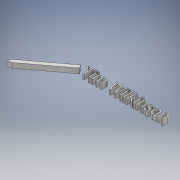
# Autodesk Inventor part: Tim
Saved by Autodesk Inventor 2017 (Build 210142000, 142)
## iProperties
Created: 2021-02-26
Part Number: Tim
Material: Generic
Document SubType Name: Modeling
Designer: paulg
Density: 1 g/cm^3
Appearance: Default
Author: paulg
Autodesk Inventor part; units mm, degrees
ref_plane "YZ Plane" through (0, 0, 0) normal (1, 0, 0) x (0, 1, 0)
ref_plane "XZ Plane" through (0, 0, 0) normal (0, 1, 0) x (-1, 0, 0)
ref_plane "XY Plane" through (0, 0, 0) normal (0, 0, 1) x (1, 0, 0)
sketch "Sketch1" plane through (0, 0, 0) normal (0, 0, 1) x (1, 0, 0)
  line L0 (-0.0217, 0.1086) -> (95.9171, 0.1086) construction
  line L1 (95.9171, 0.1086) -> (95.9171, -3.6211) construction
  line L2 (95.9171, -3.6211) -> (-0.0217, -3.6211) construction
  line L3 (-0.0217, -3.6211) -> (-0.0217, 0.1086) construction
  line L4 (-41.7116, -36.1087) -> (-2.9577, -7.16)
  line L5 (-2.9577, -7.16) -> (-5.3043, -4.0186)
  line L6 (-5.3043, -4.0186) -> (-44.0582, -32.9673)
  line L7 (-44.0582, -32.9673) -> (-41.7116, -36.1087)
  line L8 (-41.7116, -36.1087) -> (-5.3043, -4.0186) construction
  line L9 (-2.9577, -7.16) -> (-44.0582, -32.9673) construction
  line L10 (-44.0582, -32.9673) -> (-46.1916, -37.008)
  line L11 (-46.1916, -37.008) -> (-41.7116, -36.1087)
  line L12 (-46.1916, -37.008) -> (-42.8849, -34.538) construction
  line L13 (3.3251, -10.3371) -> (3.3251, -1.5202)
  line L14 (3.3251, -1.5202) -> (-0.0298, -1.5202)
  line L15 (-0.0298, -1.5202) -> (-0.0298, -0.3371)
  line L16 (-0.0298, -0.3371) -> (8.0091, -0.3371)
  line L17 (8.0091, -0.3371) -> (8.0091, -1.5202)
  line L18 (8.0091, -1.5202) -> (4.6541, -1.5202)
  line L19 (4.6541, -1.5202) -> (4.6541, -10.3371)
  line L20 (4.6541, -10.3371) -> (3.3251, -10.3371)
  line L21 (10.2133, -10.3371) -> (8.9491, -10.3371)
  line L22 (8.9491, -10.3371) -> (8.9491, -2.833)
  line L23 (8.9491, -2.833) -> (10.2133, -2.833)
  line L24 (10.2133, -2.833) -> (10.2133, -10.3371)
  line L25 (10.3024, -1.585) -> (8.8681, -1.585)
  line L26 (8.8681, -1.585) -> (8.8681, -0.2722)
  line L27 (8.8681, -0.2722) -> (10.3024, -0.2722)
  line L28 (10.3024, -0.2722) -> (10.3024, -1.585)
  line L29 (20.5779, -10.3371) -> (20.5779, -5.9935)
  spline S0 degree 2 poles (20.5779, -5.9935) (20.5779, -5.4748) (20.4969, -4.5915) (20.3672, -4.3484) knots 0 0 0 1 2 2 2
  spline S1 degree 2 poles (20.3672, -4.3484) (20.2376, -4.081) (19.7433, -3.8217) (19.3138, -3.8217) knots 0 0 0 1 2 2 2
  spline S2 degree 2 poles (19.3138, -3.8217) (18.9248, -3.8217) (18.0334, -4.2998) (17.5634, -4.7536) knots 0 0 0 1 2 2 2
  spline S3 degree 2 poles (17.5634, -4.7536) (17.5715, -4.867) (17.5877, -5.1831) (17.5877, -5.3938) knots 0 0 0 1 2 2 2
  line L30 (17.5877, -5.3938) -> (17.5877, -10.3371)
  line L31 (17.5877, -10.3371) -> (16.3235, -10.3371)
  line L32 (16.3235, -10.3371) -> (16.3235, -5.9935)
  spline S4 degree 2 poles (16.3235, -5.9935) (16.3235, -5.4748) (16.2425, -4.5915) (16.1128, -4.3484) knots 0 0 0 1 2 2 2
  spline S5 degree 2 poles (16.1128, -4.3484) (15.9831, -4.081) (15.4888, -3.8217) (15.0593, -3.8217) knots 0 0 0 1 2 2 2
  spline S6 degree 2 poles (15.0593, -3.8217) (14.6541, -3.8217) (13.7546, -4.3322) (13.3332, -4.7293) knots 0 0 0 1 2 2 2
  line L33 (13.3332, -4.7293) -> (13.3332, -10.3371)
  line L34 (13.3332, -10.3371) -> (12.069, -10.3371)
  line L35 (12.069, -10.3371) -> (12.069, -2.833)
  line L36 (12.069, -2.833) -> (13.3332, -2.833)
  line L37 (13.3332, -2.833) -> (13.3332, -3.6596)
  spline S7 degree 2 poles (13.3332, -3.6596) (13.8275, -3.1653) (14.8, -2.6223) (15.3835, -2.6223) knots 0 0 0 1 2 2 2
  spline S8 degree 2 poles (15.3835, -2.6223) (16.048, -2.6223) (17.0771, -3.2301) (17.3446, -3.9189) knots 0 0 0 1 2 2 2
  spline S9 degree 2 poles (17.3446, -3.9189) (17.9199, -3.2787) (19.0058, -2.6223) (19.6379, -2.6223) knots 0 0 0 1 2 2 2
  spline S10 degree 2 poles (19.6379, -2.6223) (20.1241, -2.6223) (20.9183, -2.9221) (21.21, -3.2625) knots 0 0 0 1 2 2 2
  spline S11 degree 2 poles (21.21, -3.2625) (21.5099, -3.6029) (21.8421, -4.6239) (21.8421, -5.3938) knots 0 0 0 1 2 2 2
  line L38 (21.8421, -5.3938) -> (21.8421, -10.3371)
  line L39 (21.8421, -10.3371) -> (20.5779, -10.3371)
  line L40 (39.2165, -0.3371) -> (36.7044, -10.3371)
  line L41 (36.7044, -10.3371) -> (35.2133, -10.3371)
  line L42 (35.2133, -10.3371) -> (33.1792, -2.0388)
  line L43 (33.1792, -2.0388) -> (31.2019, -10.3371)
  line L44 (31.2019, -10.3371) -> (29.7271, -10.3371)
  line L45 (29.7271, -10.3371) -> (27.1744, -0.3371)
  line L46 (27.1744, -0.3371) -> (28.5439, -0.3371)
  line L47 (28.5439, -0.3371) -> (30.5536, -8.6272)
  line L48 (30.5536, -8.6272) -> (32.5472, -0.3371)
  line L49 (32.5472, -0.3371) -> (33.9005, -0.3371)
  line L50 (33.9005, -0.3371) -> (35.9102, -8.7244)
  line L51 (35.9102, -8.7244) -> (37.9118, -0.3371)
  line L52 (37.9118, -0.3371) -> (39.2165, -0.3371)
  line L53 (41.599, -10.3371) -> (40.3348, -10.3371)
  line L54 (40.3348, -10.3371) -> (40.3348, -2.833)
  line L55 (40.3348, -2.833) -> (41.599, -2.833)
  line L56 (41.599, -2.833) -> (41.599, -10.3371)
  line L57 (41.6882, -1.585) -> (40.2538, -1.585)
  line L58 (40.2538, -1.585) -> (40.2538, -0.2722)
  line L59 (40.2538, -0.2722) -> (41.6882, -0.2722)
  line L60 (41.6882, -0.2722) -> (41.6882, -1.585)
  line L61 (44.7433, -10.3371) -> (43.4791, -10.3371)
  line L62 (43.4791, -10.3371) -> (43.4791, 0.1086)
  line L63 (43.4791, 0.1086) -> (44.7433, 0.1086)
  line L64 (44.7433, 0.1086) -> (44.7433, -10.3371)
  line L65 (52.8146, -10.3371) -> (51.1533, -10.3371)
  line L66 (51.1533, -10.3371) -> (48.3656, -6.7147)
  line L67 (48.3656, -6.7147) -> (47.8632, -7.2009)
  line L68 (47.8632, -7.2009) -> (47.8632, -10.3371)
  line L69 (47.8632, -10.3371) -> (46.599, -10.3371)
  line L70 (46.599, -10.3371) -> (46.599, 0.1086)
  line L71 (46.599, 0.1086) -> (47.8632, 0.1086)
  line L72 (47.8632, 0.1086) -> (47.8632, -6.0016)
  line L73 (47.8632, -6.0016) -> (50.8292, -2.833)
  line L74 (50.8292, -2.833) -> (52.4013, -2.833)
  line L75 (52.4013, -2.833) -> (49.3219, -5.9692)
  line L76 (49.3219, -5.9692) -> (52.8146, -10.3371)
  line L77 (54.7352, -10.3371) -> (53.471, -10.3371)
  line L78 (53.471, -10.3371) -> (53.471, -2.833)
  line L79 (53.471, -2.833) -> (54.7352, -2.833)
  line L80 (54.7352, -2.833) -> (54.7352, -10.3371)
  line L81 (54.8243, -1.585) -> (53.3899, -1.585)
  line L82 (53.3899, -1.585) -> (53.3899, -0.2722)
  line L83 (53.3899, -0.2722) -> (54.8243, -0.2722)
  line L84 (54.8243, -0.2722) -> (54.8243, -1.585)
  line L85 (62.4823, -10.3371) -> (61.2181, -10.3371)
  line L86 (61.2181, -10.3371) -> (61.2181, -6.0583)
  spline S12 degree 2 poles (61.2181, -6.0583) (61.2181, -5.5397) (61.1209, -4.6482) (60.975, -4.3808) knots 0 0 0 1 2 2 2
  spline S13 degree 2 poles (60.975, -4.3808) (60.8211, -4.0972) (60.27, -3.8217) (59.8, -3.8217) knots 0 0 0 1 2 2 2
  spline S14 degree 2 poles (59.8, -3.8217) (59.33, -3.8217) (58.3332, -4.3241) (57.8551, -4.7293) knots 0 0 0 1 2 2 2
  line L87 (57.8551, -4.7293) -> (57.8551, -10.3371)
  line L88 (57.8551, -10.3371) -> (56.5909, -10.3371)
  line L89 (56.5909, -10.3371) -> (56.5909, -2.833)
  line L90 (56.5909, -2.833) -> (57.8551, -2.833)
  line L91 (57.8551, -2.833) -> (57.8551, -3.6677)
  spline S15 degree 2 poles (57.8551, -3.6677) (58.4224, -3.1572) (59.5164, -2.6223) (60.1322, -2.6223) knots 0 0 0 1 2 2 2
  spline S16 degree 2 poles (60.1322, -2.6223) (61.2343, -2.6223) (62.4823, -4.081) (62.4823, -5.4667) knots 0 0 0 1 2 2 2
  line L92 (62.4823, -5.4667) -> (62.4823, -10.3371)
  spline S17 degree 2 poles (66.283, -10.5153) (65.5293, -10.5153) (64.2246, -10.1102) (63.7951, -9.8833) knots 0 0 0 1 2 2 2
  line L93 (63.7951, -9.8833) -> (63.7951, -8.4651)
  line L94 (63.7951, -8.4651) -> (63.86, -8.4651)
  spline S18 degree 2 poles (63.86, -8.4651) (64.022, -8.5948) (64.4596, -8.9027) (64.8243, -9.0729) knots 0 0 0 1 2 2 2
  spline S19 degree 2 poles (64.8243, -9.0729) (65.1403, -9.2268) (65.9183, -9.4538) (66.3316, -9.4538) knots 0 0 0 1 2 2 2
  spline S20 degree 2 poles (66.3316, -9.4538) (66.6314, -9.4538) (67.3202, -9.316) (67.4823, -9.2025) knots 0 0 0 1 2 2 2
  spline S21 degree 2 poles (67.4823, -9.2025) (67.7173, -9.0486) (67.928, -8.7001) (67.928, -8.3435) knots 0 0 0 1 2 2 2
  spline S22 degree 2 poles (67.928, -8.3435) (67.928, -7.8978) (67.4418, -7.4359) (66.8178, -7.282) knots 0 0 0 1 2 2 2
  spline S23 degree 2 poles (66.8178, -7.282) (66.5747, -7.2252) (65.7967, -7.0632) (65.4645, -6.974) knots 0 0 0 1 2 2 2
  spline S24 degree 2 poles (65.4645, -6.974) (64.6055, -6.7228) (63.8275, -5.6855) (63.8275, -4.9481) knots 0 0 0 1 2 2 2
  spline S25 degree 2 poles (63.8275, -4.9481) (63.8275, -3.927) (65.3591, -2.6547) (66.6233, -2.6547) knots 0 0 0 1 2 2 2
  spline S26 degree 2 poles (66.6233, -2.6547) (67.2473, -2.6547) (68.5115, -2.9627) (68.941, -3.1977) knots 0 0 0 1 2 2 2
  line L95 (68.941, -3.1977) -> (68.941, -4.551)
  line L96 (68.941, -4.551) -> (68.8762, -4.551)
  spline S27 degree 2 poles (68.8762, -4.551) (68.3899, -4.162) (67.2068, -3.7163) (66.599, -3.7163) knots 0 0 0 1 2 2 2
  spline S28 degree 2 poles (66.599, -3.7163) (65.975, -3.7163) (65.116, -4.2431) (65.116, -4.7698) knots 0 0 0 1 2 2 2
  spline S29 degree 2 poles (65.116, -4.7698) (65.116, -5.2479) (65.6266, -5.7098) (66.1938, -5.8557) knots 0 0 0 1 2 2 2
  spline S30 degree 2 poles (66.1938, -5.8557) (66.4694, -5.9286) (67.1663, -6.0745) (67.5472, -6.1636) knots 0 0 0 1 2 2 2
  spline S31 degree 2 poles (67.5472, -6.1636) (68.3737, -6.3743) (69.2165, -7.3387) (69.2165, -8.1734) knots 0 0 0 1 2 2 2
  spline S32 degree 2 poles (69.2165, -8.1734) (69.2165, -8.6596) (68.8356, -9.5186) (68.4629, -9.8346) knots 0 0 0 1 2 2 2
  spline S33 degree 2 poles (68.4629, -9.8346) (68.0658, -10.1669) (67.0528, -10.5153) (66.283, -10.5153) knots 0 0 0 1 2 2 2
  spline S34 degree 2 poles (76.5585, -6.585) (76.5585, -8.4813) (74.7352, -10.5478) (73.2117, -10.5478) knots 0 0 0 1 2 2 2
  spline S35 degree 2 poles (73.2117, -10.5478) (71.6476, -10.5478) (69.8567, -8.4165) (69.8567, -6.585) knots 0 0 0 1 2 2 2
  spline S36 degree 2 poles (69.8567, -6.585) (69.8567, -4.705) (71.7044, -2.6223) (73.2117, -2.6223) knots 0 0 0 1 2 2 2
  spline S37 degree 2 poles (73.2117, -2.6223) (74.7352, -2.6223) (76.5585, -4.6969) (76.5585, -6.585) knots 0 0 0 1 2 2 2
  spline S38 degree 2 poles (75.2538, -6.585) (75.2538, -5.1264) (74.1922, -3.7082) (73.2117, -3.7082) knots 0 0 0 1 2 2 2
  spline S39 degree 2 poles (73.2117, -3.7082) (72.2311, -3.7082) (71.1614, -5.1264) (71.1614, -6.585) knots 0 0 0 1 2 2 2
  spline S40 degree 2 poles (71.1614, -6.585) (71.1614, -8.0032) (72.2311, -9.4619) (73.2117, -9.4619) knots 0 0 0 1 2 2 2
  spline S41 degree 2 poles (73.2117, -9.4619) (74.1841, -9.4619) (75.2538, -8.0275) (75.2538, -6.585) knots 0 0 0 1 2 2 2
  line L97 (83.7465, -10.3371) -> (82.4823, -10.3371)
  line L98 (82.4823, -10.3371) -> (82.4823, -6.0583)
  spline S42 degree 2 poles (82.4823, -6.0583) (82.4823, -5.5397) (82.3851, -4.6482) (82.2392, -4.3808) knots 0 0 0 1 2 2 2
  spline S43 degree 2 poles (82.2392, -4.3808) (82.0852, -4.0972) (81.5342, -3.8217) (81.0642, -3.8217) knots 0 0 0 1 2 2 2
  spline S44 degree 2 poles (81.0642, -3.8217) (80.5942, -3.8217) (79.5974, -4.3241) (79.1193, -4.7293) knots 0 0 0 1 2 2 2
  line L99 (79.1193, -4.7293) -> (79.1193, -10.3371)
  line L100 (79.1193, -10.3371) -> (77.8551, -10.3371)
  line L101 (77.8551, -10.3371) -> (77.8551, -2.833)
  line L102 (77.8551, -2.833) -> (79.1193, -2.833)
  line L103 (79.1193, -2.833) -> (79.1193, -3.6677)
  spline S45 degree 2 poles (79.1193, -3.6677) (79.6865, -3.1572) (80.7805, -2.6223) (81.3964, -2.6223) knots 0 0 0 1 2 2 2
  spline S46 degree 2 poles (81.3964, -2.6223) (82.4985, -2.6223) (83.7465, -4.081) (83.7465, -5.4667) knots 0 0 0 1 2 2 2
  line L104 (83.7465, -5.4667) -> (83.7465, -10.3371)
  point P0 (0, 0)
  point P1 (-23.5079, -20.0636)
  constraints: 18 end point, 3 midpoint, 3 parallel, 1 perpendicular, 2 other
extrude "Extrusion1" add sketch "Sketch1" along normal blind 5
body "Solid1"
